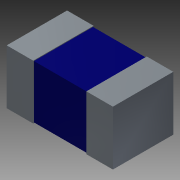
# Autodesk Inventor part: 0603_cap
Saved by Autodesk Inventor 2013 (Build 170138000, 138)
## iProperties
Created: 2015-06-30
Part Number: 0603_cap
Material: Ogólny
Document SubType Name: Modeling
Designer: terg
Density: 1 g/cm^3
Author: terg
Autodesk Inventor part; units mm, degrees
ref_plane "YZ Plane" through (0, 0, 0) normal (1, 0, 0) x (0, 1, 0)
ref_plane "XZ Plane" through (0, 0, 0) normal (0, 1, 0) x (-1, 0, 0)
ref_plane "XY Plane" through (0, 0, 0) normal (0, 0, 1) x (1, 0, 0)
sketch "Szkic1" plane through (0, 0, 0) normal (0, 1, 0) x (-1, 0, 0)
  line L0 (0, 0) -> (1.6, 0)
  line L1 (1.6, 0) -> (1.6, 0.8)
  line L2 (1.6, 0.8) -> (0, 0.8)
  line L3 (0, 0.8) -> (0, 0)
  dimension "d0" = 1.6
  dimension "d1" = 0.8
  constraints: 8 end point, 2 parallel, 1 horizontal, 1 perpendicular
  measures "d0" distance of L2.end L1.end
  measures "d1" distance of L1.end L0.end
extrude "Wyciągnięcie proste1" add sketch "Szkic1" along normal blind 0.89
sketch "Szkic2" plane through (0, 0.89, 0) normal (0, 1, 0) x (1, 0, 0)
  line L0 (-1.6, 0) -> (-1.2, 0)
  line L1 (-1.2, 0) -> (-1.2, -0.8)
  line L2 (-1.2, -0.8) -> (-1.6, -0.8)
  line L3 (-1.6, -0.8) -> (-1.6, 0)
  line L4 (0, 0) -> (-0.4, 0)
  line L5 (-0.4, 0) -> (-0.4, -0.8)
  line L6 (-0.4, -0.8) -> (0, -0.8)
  line L7 (0, -0.8) -> (0, 0)
  dimension "d4" = 0.4
  dimension "d5" = 0.8
  dimension "d6" = 0.4
  dimension "d7" = 0.8
  constraints: 16 end point, 4 parallel, 2 horizontal, 2 perpendicular
  measures "d4" distance of L1.end L2.end
  measures "d5" distance of L0.end L1.end
  measures "d6" distance of L6.end L5.end
  measures "d7" distance of L5.end L4.end
extrude "Wyciągnięcie proste2" add sketch "Szkic2" along normal blind 0.01 and the other way blind 0.9
sketch "Szkic4" plane through (-1.2, 0, 0.8) normal (0, 0, 1) x (1, 0, 0)
  line L0 (-0.4, -0.01) -> (-0.4, 0.9) projected
  line L1 (0, -0.01) -> (-0.4, -0.01) projected
  line L2 (-0.4, 0.9) -> (0, 0.9)
  line L3 (0, 0.9) -> (0, -0.01)
  line L4 (0, -0.01) -> (-0.4, -0.01)
  line L5 (-0.4, -0.01) -> (-0.4, 0.9)
  line L6 (1.2, 0.9) -> (0.8, 0.9)
  line L7 (0.8, 0.9) -> (0.8, -0.01)
  line L8 (0.8, -0.01) -> (1.2, -0.01)
  line L9 (1.2, -0.01) -> (1.2, 0.9)
  point P0 (1.2, 0)
  point P1 (-0.5, 0)
  constraints: 16 end point, 4 parallel, 2 horizontal, 2 perpendicular, 1 other
extrude "Wyciągnięcie proste3" add sketch "Szkic4" along normal blind 0.01 and the other way blind 0.81
